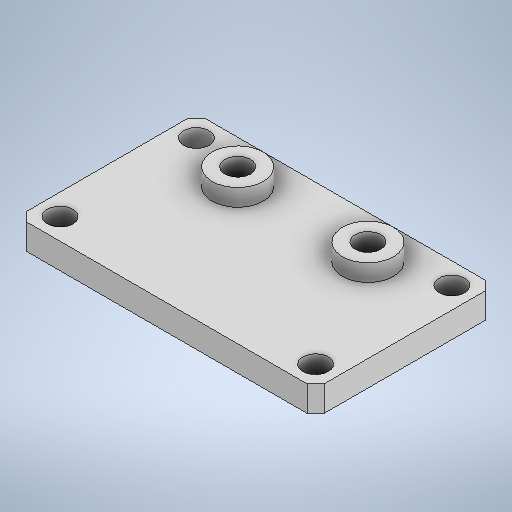
# Autodesk Inventor part: Sensor
Saved by Autodesk Inventor 2025 (Build 290162000, 162)
## iProperties
Created: 2025-04-09
Part Number: Sensor
Material: Genérico
Document SubType Name: Modeling
Designer: Ian
Density: 1 g/cm^3
Appearance: Padrão
Author: Ian
Autodesk Inventor part; units mm, degrees
ref_plane "YZ Plane" through (0, 0, 0) normal (1, 0, 0) x (0, 1, 0)
ref_plane "XZ Plane" through (0, 0, 0) normal (0, 1, 0) x (-1, 0, 0)
ref_plane "XY Plane" through (0, 0, 0) normal (0, 0, 1) x (1, 0, 0)
sketch "Esboço1" plane through (0, 0, 0) normal (0, 1, 0) x (-1, 0, 0)
  line L0 (-17.5, 10.5) -> (17.5, 10.5)
  line L1 (17.5, 10.5) -> (17.5, -10.5)
  line L2 (17.5, -10.5) -> (-17.5, -10.5)
  line L3 (-17.5, -10.5) -> (-17.5, 10.5)
  line L4 (-17.5, 10.5) -> (17.5, -10.5) construction
  line L5 (17.5, 10.5) -> (-17.5, -10.5) construction
  point P0 (0, 0)
  point P1 (0, 0)
  dimension "d1" = 35
  dimension "d29" = 21
  constraints: 12 end point, 2 midpoint, 2 parallel, 1 coincident, 1 horizontal, 1 perpendicular, 1 other
  measures "d1" distance of L1.end L2.end
  measures "d29" distance of L0.end L1.end
extrude "Extrusão1" add sketch "Esboço1" along normal blind 3
sketch "Esboço2" plane through (0, 3, 0) normal (0, 1, 0) x (1, 0, 0)
  line L0 (-17.5, -10.5) -> (17.5, -10.5) projected
  line L1 (-17.5, 10.5) -> (-17.5, -10.5) projected
  line L2 (-17.5, 0) -> (-17.5, 9.5148)
  line L3 (-17.5, 0) -> (-17.5, 10.5)
  line L4 (17.5, -10.5) -> (17.5, 10.5) projected
  circle A0 centre (7.65, 5.5) radius 1.5
  circle A1 centre (7.65, 5.5) radius 3
  circle A2 centre (-7.65, 5.5) radius 1.5
  circle A3 centre (-7.65, 5.5) radius 3
  line L5 (17.5, 10.5) -> (-17.5, 10.5) projected
  line L6 (-17.5, 5.5) -> (17.5, 5.5)
  dimension "d50" = 3
  dimension "d51" = 6
  dimension "d63" = 3
  dimension "d64" = 6
  dimension "d65" = 15.3
  dimension "d78" = 5
  constraints: 6 end point, 5 point on line, 4 centre point, 2 coincident, 1 midpoint, 1 perpendicular
  measures "d50" diameter of A0
  measures "d51" diameter of A1
  measures "d63" diameter of A2
  measures "d64" diameter of A3
  measures "d65" distance of A0.centre A2.centre
  measures "d78" distance between parallel lines of L6 L5
extrude "Extrusão2" add sketch "Esboço2" along normal blind 2 contours L6 A0 A1 | A1 L6 A0 | L6 A2 A3 | A3 L6 A2
sketch "Esboço5" plane through (0, 3, 0) normal (0, 1, 0) x (1, 0, 0)
  circle A0 centre (-15, -8) radius 1.5
  circle A1 centre (-15, 8) radius 1.5
  circle A2 centre (15, -8) radius 1.5
  circle A3 centre (15, 8) radius 1.5
  line L0 (17.5, 10.5) -> (-17.5, 10.5) projected
  line L1 (17.5, -10.5) -> (17.5, 10.5) projected
  line L2 (-17.5, -10.5) -> (17.5, -10.5) projected
  line L3 (-17.5, 10.5) -> (-17.5, -10.5) projected
  point P0 (0, 0)
  dimension "d32" = 3
  dimension "d33" = 2.5
  dimension "d34" = 2.5
  dimension "d35" = 2.5
  dimension "d36" = 2.5
  dimension "d37" = 2.5
  dimension "d38" = 2.5
  dimension "d39" = 2.5
  dimension "d40" = 2.5
  constraints: 4 centre point, 3 equal radius
  measures "d32" diameter of A0
  measures "d33" distance from line of L0 A3.centre
  measures "d34" distance from line of A3.centre L1
  measures "d35" distance from line of L1 A2.centre
  measures "d36" distance from line of L2 A2.centre
  measures "d37" distance from line of L3 A0.centre
  measures "d38" distance from line of L2 A0.centre
  measures "d39" distance from line of L3 A1.centre
  measures "d40" distance from line of L0 A1.centre
extrude "Extrusão4" cut sketch "Esboço5" against normal through all contours A0 | A1 | A2 | A3
chamfer "Chanfro1" distance 1 angle 45 4 edges at (-17.5, 1.5, 10.5) (-17.5, 1.5, -10.5) (17.5, 1.5, 10.5) (17.5, 1.5, -10.5)
sketch "Esboço6" plane through (7.65, 5, -5.5) normal (0, 1, 0) x (1, 0, 0)
  circle A0 centre (0, 0) radius 1.5
  circle A1 centre (-15.3, 0) radius 3 projected
  circle A2 centre (-15.3, 0) radius 1.5 projected
  circle A3 centre (-15.3, 0) radius 1.5
  point P0 (-7.65, -5.5)
  constraints: 2 centre point, 1 coincident, 1 concentric
extrude "Extrusão5" cut sketch "Esboço6" against normal through all contours A0 | A2
